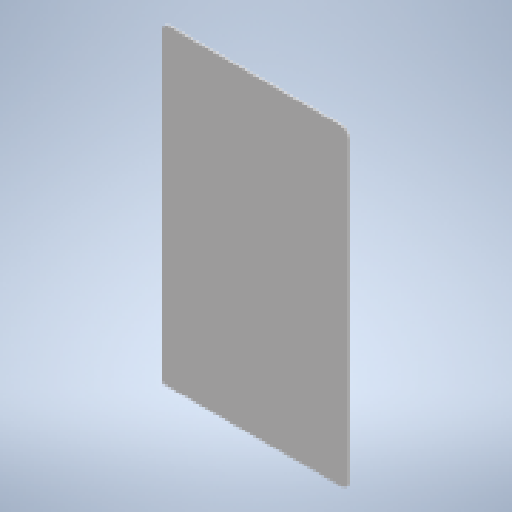
# Autodesk Inventor part: Side Stiffener
Saved by Autodesk Inventor 2025 (Build 290162000, 162)
## iProperties
Created: 2024-11-12
Part Number: Side Stiffener
Material: Generic
Document SubType Name: Modeling
Designer: Caleb Fangmeier
Density: 1 g/cm^3
Appearance: Default
Author: Caleb Fangmeier
Autodesk Inventor part; units mm, degrees
ref_plane "YZ Plane" through (0, 0, 0) normal (1, 0, 0) x (0, 1, 0)
ref_plane "XZ Plane" through (0, 0, 0) normal (0, 1, 0) x (-1, 0, 0)
ref_plane "XY Plane" through (0, 0, 0) normal (0, 0, 1) x (1, 0, 0)
sketch "Sketch1" plane through (0, 0, 0) normal (0, 0, 1) x (1, 0, 0)
  line L0 (-139.8225, -42.851) -> (-139.8018, -82.2454) projected
  arc A0 (-138.8232, -41.8607) -> (-139.8225, -42.851) centre (-138.8223, -42.8609) ccw projected
  line L1 (-116.3009, -41.8403) -> (-138.8232, -41.8607) projected
  arc A1 (-115.3058, -42.8403) -> (-116.3009, -41.8403) centre (-116.306, -42.8405) ccw projected
  line L2 (-115.2978, -81.8628) -> (-115.3058, -42.8403) projected
  arc A2 (-116.299, -82.8549) -> (-115.2978, -81.8628) centre (-116.2978, -81.8549) ccw projected
  arc A3 (-139.8018, -82.2454) -> (-139.3074, -83.1072) centre (-138.8025, -82.2449) ccw projected
  line L3 (-116.0766, -82.8302) -> (-139.5966, -82.8514)
  circle A4 centre (-131.3626, -67.5261) radius 1.1 projected
  circle A5 centre (-135.8392, -58.9026) radius 1.1 projected
  point P0 (0, 0)
  dimension "d0" = 40.99
  constraints: 2 end point, 2 point on circle, 1 parallel
  measures "d0" distance between parallel lines of L1 L3
extrude "Extrusion1" add sketch "Sketch1" along normal blind 0.2
body "Solid1"
